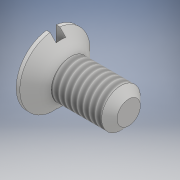
# Autodesk Inventor part: винт
Saved by Autodesk Inventor 2018 (Build 220112000, 112)
## iProperties
Created: 2018-05-24
Part Number: винт
Material: Типовые
Document SubType Name: Modeling
Designer: user
Density: 1 g/cm^3
Appearance: По умолчанию
Author: user
Autodesk Inventor part; units mm, degrees
ref_plane "YZ Plane" through (0, 0, 0) normal (1, 0, 0) x (0, 1, 0)
ref_plane "XZ Plane" through (0, 0, 0) normal (0, 1, 0) x (-1, 0, 0)
ref_plane "XY Plane" through (0, 0, 0) normal (0, 0, 1) x (1, 0, 0)
sketch "Эскиз1" plane through (0, 0, 0) normal (1, 0, 0) x (0, 1, 0)
  circle A0 centre (0, 0) radius 4
  dimension "d0" = 8
  constraints: 1 centre point, 1 coincident
  measures "d0" diameter of A0
extrude "Выдавливание1" add sketch "Эскиз1" along normal blind 12
chamfer "Фаска1" distance 1.6 angle 45 1 edges at (12, -4, 0)
thread "Резьба1" size "M8x1.25" class "6g" standard "ANSI Metric M Profile" full length
sketch "Эскиз2" plane through (0, 0, 0) normal (0, 0, 1) x (1, 0, 0)
  line L0 (0, 4) -> (0, -4) projected
  line L1 (0, 0) -> (0, 4)
  line L2 (0, 4) -> (-4, 8)
  line L3 (0, 4) -> (5.6569, 4) construction
  line L4 (-4, 8) -> (-4, 4)
  line L5 (-4, 0) -> (0, 0)
  line L6 (0, 4) -> (0, 0)
  line L7 (-4, 0) -> (-4, 4)
  dimension "d8" = 4
  dimension "d9" = 135
  constraints: 14 end point, 2 collinear, 1 equal length, 1 horizontal, 1 perpendicular, 1 point on line, 1 vertical
  measures "d8" distance of L0.start L4.end
  measures "d9" angle of L3 L2
revolve "Вращение1" add sketch "Эскиз2" angle 360 about axis through (-4, 0, 0) along (1, 0, 0)
sketch "Эскиз3" plane through (-4, 0, 0) normal (-1, 0, 0) x (0, 0, 1)
  circle A0 centre (0, 0) radius 7.25
  dimension "d11" = 14.5
  constraints: 1 centre point, 1 coincident
  measures "d11" diameter of A0
extrude "Выдавливание2" cut sketch "Эскиз3" against normal blind 25.25 keep common part
sketch "Эскиз4" plane through (0, 0, 0) normal (0, 0, 1) x (1, 0, 0)
  line L0 (-6, 1) -> (-2, 1)
  line L1 (-2, 1) -> (-2, -1)
  line L2 (-2, -1) -> (-6, -1)
  line L3 (-6, -1) -> (-6, 1)
  line L4 (-4, -7.25) -> (-4, 7.25) projected
  line L5 (-6, 1) -> (-2, -1) construction
  line L6 (-2, 1) -> (-6, -1) construction
  point P0 (0, 0)
  point P1 (-4, 0)
  dimension "d14" = 4
  dimension "d15" = 2
  constraints: 12 end point, 3 midpoint, 2 parallel, 1 horizontal, 1 perpendicular
  measures "d14" distance of L1.end L2.end
  measures "d15" distance of L0.end L1.end
extrude "Выдавливание3" cut sketch "Эскиз4" along normal mid plane 25.25
